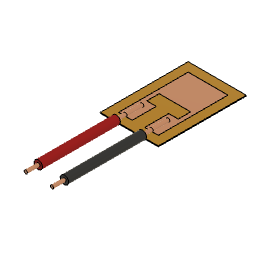
BF120-2AA (Autodesk Fusion 360 design; units mm, degrees)
Autodesk Fusion 360 part; units mm, degrees
note: some values were not read from the file. Set by a fixed rule: which sketch regions a step uses.
sketch "Sketch1" plane through (0, 0, 0) normal (0, 0, 1) x (1, 0, 0)
  line L0 (1.75, -2.65) -> (-1.75, -2.65)
  line L1 (-1.75, -2.65) -> (-1.75, 2.65)
  line L2 (-1.75, 2.65) -> (1.75, 2.65)
  line L3 (1.75, 2.65) -> (1.75, -2.65)
  line L4 (1.75, -2.65) -> (-1.75, 2.65) construction
  line L5 (-1.75, -2.65) -> (1.75, 2.65) construction
  line L6 (-1.2, 0.1) -> (-1.2, 2.1)
  line L7 (-1.2, 2.1) -> (1.2, 2.1)
  line L8 (1.2, 2.1) -> (1.2, 0.1)
  line L9 (1.2, 0.1) -> (-1.2, 2.1) construction
  line L10 (-1.2, 0.1) -> (1.2, 2.1) construction
  line L11 (0, 0) -> (0, 1.1)
  line L12 (-1.75, -3.4) -> (1.75, -3.4) construction
  line L13 (1.75, -3.4) -> (1.75, -2.65) construction
  line L14 (1.75, -2.65) -> (-1.75, -2.65) construction
  line L15 (-1.75, -2.65) -> (-1.75, -3.4) construction
  line L16 (-1.2, 0.1) -> (-1.2, -2.1)
  line L17 (-1.2, -2.1) -> (-0.375, -2.1)
  line L18 (-0.375, -2.1) -> (-0.375, -0.65)
  line L19 (-0.375, -0.65) -> (-0.95, -0.65)
  line L20 (-0.95, -0.65) -> (-0.95, 0.1)
  line L21 (1.2, 0.1) -> (1.2, -2.1)
  line L22 (1.2, -2.1) -> (0.375, -2.1)
  line L23 (0.375, -2.1) -> (0.375, -0.65)
  line L24 (0.375, -0.65) -> (0.95, -0.65)
  line L25 (0.95, -0.65) -> (0.95, 0.1)
  line L26 (-0.95, 0.1) -> (0.95, 0.1)
  line L27 (-0.7875, -8.1) -> (-0.8884, -8.1)
  line L28 (-0.8884, -8.1) -> (-0.8884, -2.1)
  line L29 (-0.7875, -2.1) -> (-0.7875, -8.1)
  line L30 (-0.7875, -8.1) -> (-1.0384, -8.1)
  line L31 (-1.0384, -8.1) -> (-1.0384, -2.1)
  line L32 (1.0384, -8.1) -> (1.0384, -2.1)
  line L33 (1.0384, -2.1) -> (0.7875, -2.1)
  line L34 (0.7875, -2.1) -> (0.7875, -8.1)
  line L35 (0.7875, -8.1) -> (1.0384, -8.1)
  line L36 (0.8884, -8.1) -> (0.8884, -2.1)
  line L37 (-1.0384, -7.35) -> (-0.8884, -7.35)
  line L38 (1.0384, -7.35) -> (0.8884, -7.35)
  line L39 (-0.8884, -2.1) -> (-0.8926, -1.1)
  line L40 (-0.7875, -1.0996) -> (-0.7875, -2.1)
  line L41 (-0.7875, -1.0996) -> (-0.8926, -1.1)
  line L42 (0.8884, -2.1) -> (0.8926, -1.1)
  line L43 (0.7875, -1.0996) -> (0.8926, -1.1)
  line L44 (0.7875, -1.0996) -> (0.7875, -2.1)
  point P0 (0, 1.1)
  dimension "d3" = 3.5
  dimension "d4" = 5.3
  dimension "d5" = 2.4
  dimension "d7" = 0.55
  dimension "d8" = 0.55
  dimension "d9" = 0.55
  dimension "d10" = 0.25
  dimension "d12" = 0.75
  dimension "d13" = 0.25
  dimension "d17" = 0.55
  dimension "d20" = 0.75
  dimension "d21" = 2
  dimension "d22" = 0.75
  dimension "d27" = 0.1009
  dimension "d28" = 6
  dimension "d30" = 0.15
  dimension "d33" = 0.75
  dimension "d36" = 1
  constraint coincident L11.start origin
  constraint horizontal L0
  constraint perpendicular L0 L1
  constraint parallel L0 L2
  constraint parallel L1 L3
  constraint coincident L4 L11.start
  constraint coincident L5 L11.start
  constraint parallel L6 L8
  constraint coincident L9 P0
  constraint coincident L10 P0
  constraint vertical L11
  constraint coincident P0 L11.end
  constraint coincident L0.end
  constraint coincident L0.start
  constraint perpendicular L16 L17
  constraint perpendicular L17 L18
  constraint perpendicular L18 L19
  constraint symmetric L6.start L11 L8.end
  constraint symmetric L11 L16.end L21.end
  constraint symmetric L11 L17.end L22.end
  constraint symmetric L11 L18.end L23.end
  constraint symmetric L11 L19.end L24.end
  constraint symmetric L11 L20.end L25.end
  constraint horizontal L27
  constraint vertical L28
  constraint vertical L29
  constraint horizontal L30
  constraint vertical L31
  constraint coincident L27.start L29
  constraint coincident L40.end L29
  constraint coincident L27.end L30
  constraint midpoint L17 L29.start
  constraint symmetric L11 L28.end L36.end
  constraint symmetric L11 L27.end L36.start
  constraint symmetric L11 L31.end L32.end
  constraint symmetric L11 L29.start L33.end
  constraint symmetric L11 L27.start L34.end
  constraint symmetric L11 L30.end L32.start
  constraint coincident L31 L37.start
  constraint coincident L28 L37.end
  constraint perpendicular L28 L37
  constraint symmetric L11 L37.start L38.start
  constraint symmetric L11 L37.end L38.end
  constraint perpendicular L17 L40
  constraint perpendicular L39 L41
  constraint symmetric L11 L39.end L42.end
  constraint symmetric L11 L40.start L43.start
  constraint coincident L39.end L41.end
  constraint coincident L17 L31.end
  constraint vertical L8
  constraint coincident L6.start L26
  constraint coincident L8.end L9.start
  constraint coincident L29.start L40.end
  constraint coincident L17 L28.end
  measures "d3" distance of L1.end L2.end
  measures "d4" distance of L0.end L1.end
  measures "d5" distance of L6.end L7.end
  measures "d7" distance of L2 L7
  measures "d8" distance of L3 L8
  measures "d9" distance of L1 L6
  measures "d13" distance of L16 L20
  measures "d17" distance of L0 L17
  measures "d20" distance of L19 L26
  measures "d21" distance of L7 L26
  measures "d22" distance of L18 L23
  measures "d27" distance of L28.end L29.start
  measures "d28" distance of L28.end L27.end
  measures "d30" distance of L28 L31
  measures "d33" distance of L30 L37
  measures "d36" vertical distance of L28.end L39.end
extrude "Extrude1" add sketch "Sketch1" against normal blind 0.05 contours L0 L1 L2 L3 L6 L7 L8 L16 L17 L21 L22 L31 L32 | L0 L22 L32 L33 L36 | L0 L22 L33 L34 L36 | L6 L7 L8 L16 L17 L18 L19 L20 L21 L22 L23 L24 L25 L26 L33 L39 L40 L41 L42 L43 L44 | L0 L17 L18 L19 L20 L22 L23 L24 L25 L26 L29 L34 | L22 L33 L42 L43 L44 | L0 L17 L28 L29 | L0 L17 L28 L31 | L17 L39 L40 L41 makes body 1
extrude "Extrude2" add sketch "Sketch1" along normal blind 0.005 separate body contours L6 L7 L8 L16 L17 L18 L19 L20 L21 L22 L23 L24 L25 L26 L33 L39 L40 L41 L42 L43 L44 | L22 L33 L42 L43 L44 | L17 L39 L40 L41 makes body 2
revolve "Revolve1" add sketch "Sketch1" angle 360 about axis through (-0.7875, -2.1, 0) along (0, -1, 0) separate body contours L0 L27 L28 L29 L30 | L0 L17 L28 L29 | L17 L39 L40 L41 makes body 3
revolve "Revolve2" add sketch "Sketch1" angle 360 about axis through (-0.7875, -2.1, 0) along (0, -1, 0) separate body contours L0 L28 L31 L37 makes body 4
revolve "Revolve3" add sketch "Sketch1" angle 360 about axis through (0.7875, -2.1, 0) along (0, -1, 0) separate body contours L0 L34 L35 L36 | L0 L22 L33 L34 L36 | L22 L33 L42 L43 L44 makes body 5
revolve "Revolve4" add sketch "Sketch1" angle 360 about axis through (0.7875, -2.1, 0) along (0, -1, 0) separate body contours L0 L32 L36 L38 makes body 6
move_body "Move1" bodies 6 5 3 4 to x (1, 0, 0) y (0, 1, 0) z (0, 0, 1) at (0, 0, 0.101)
equation "d27 = ( 0.2019 / 2 ) * 1 mm"
